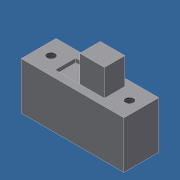
# Autodesk Inventor part: P1704_013_Switch
Saved by Autodesk Inventor 2019 (Build 230136000, 136)
## iProperties
Created: 2019-05-23
Part Number: P1704_013_Switch
Project: Nom Projet
Material: .
Description: Nom pièce
Document SubType Name: Modeling
Designer: Adel.KAHRIMANOVIC
Authority: brut Ø
Density: 0.001 g/cm^3
Appearance: Par défaut
Author: Adel.KAHRIMANOVIC
Material number: ---
Autodesk Inventor part; units mm, degrees
ref_plane "Plan YZ" through (0, 0, 0) normal (1, 0, 0) x (0, 1, 0)
ref_plane "Plan XZ" through (0, 0, 0) normal (0, 1, 0) x (-1, 0, 0)
ref_plane "Plan XY" through (0, 0, 0) normal (0, 0, 1) x (1, 0, 0)
sketch "Esquisse1" plane through (0, 0, 0) normal (0, 0, 1) x (1, 0, 0)
  line L0 (0, 0) -> (-25, 0)
  line L1 (-25, 0) -> (-25, 8.5)
  line L2 (-25, 8.5) -> (0, 8.5)
  line L3 (0, 8.5) -> (0, 0)
  dimension "d0" = 25
  dimension "d1" = 8.5
  constraints: 8 end point, 2 parallel, 1 horizontal, 1 perpendicular
  measures "d0" distance of L1.end L2.end
  measures "d1" distance between parallel lines of L0 L2
extrude "Extrusion1" add sketch "Esquisse1" along normal blind 11.5
sketch "Esquisse6" plane through (0, 0, 11.5) normal (0, 0, 1) x (1, 0, 0)
  line L0 (-18.5, 1.75) -> (-6.5, 1.75)
  line L1 (-6.5, 1.75) -> (-6.5, 6.75)
  line L2 (-6.5, 6.75) -> (-18.5, 6.75)
  line L3 (-18.5, 6.75) -> (-18.5, 1.75)
  line L4 (-6.5, 4.25) -> (0, 4.25) construction
  line L5 (0, 0) -> (0, 8.5) projected
  line L6 (-25, 4.25) -> (-18.5, 4.25) construction
  line L7 (-25, 8.5) -> (-25, 0) construction
  line L8 (-21.7955, 8.5) -> (-21.7955, 6.75) construction
  line L9 (-18.2379, 0) -> (-18.2379, 1.75) construction
  line L10 (-25, 0) -> (0, 0) construction
  line L11 (0, 8.5) -> (-25, 8.5) construction
  dimension "d4" = 5
  dimension "d5" = 12
  constraints: 16 end point, 4 midpoint, 4 point on line, 3 horizontal, 2 equal length, 2 parallel, 2 vertical, 1 collinear, 1 perpendicular
  measures "d4" distance between parallel lines of L2 L0
  measures "d5" distance of L1.end L2.end
extrude "Extrusion2" cut sketch "Esquisse6" against normal blind 1
sketch "Esquisse7" plane through (0, 0, 10.5) normal (0, 0, 1) x (1, 0, 0)
  line L0 (-6.5, 1.75) -> (-12.5, 1.75)
  line L1 (-12.5, 1.75) -> (-12.5, 6.75)
  line L2 (-12.5, 6.75) -> (-6.5, 6.75)
  line L3 (-6.5, 6.75) -> (-6.5, 1.75)
  line L4 (-6.5, 1.75) -> (-18.5, 1.75) projected
  line L5 (-18.5, 6.75) -> (-6.5, 6.75) projected
  line L6 (-6.5, 6.75) -> (-6.5, 1.75) projected
  point P0 (0, 0)
  dimension "d8" = 6
  constraints: 8 end point, 3 collinear, 2 parallel, 1 horizontal, 1 perpendicular
  measures "d8" distance of L1.end L2.end
extrude "Extrusion3" add sketch "Esquisse7" along normal blind 7.5
sketch "Esquisse8" plane through (0, 0, 11.5) normal (0, 0, 1) x (1, 0, 0)
  line L0 (-3, 4.354) -> (-3, 0.0702) construction
  line L1 (-3, 8.6378) -> (-3, 4.354) construction
  line L2 (0, 0) -> (0, 8.5) construction
  dimension "d18" = 3
  constraints: 4 end point, 2 vertical, 1 collinear
  measures "d18" distance from line of L2 L0.start
hole "Perçage1" at (-3, 4.354, 11.5) direction (0, 0, -1) diameter 2.013 end through all thread size "M2.5x0.45" class "6H" standard "ISO M"
sketch "Esquisse9" plane through (0, 0, 11.5) normal (0, 0, 1) x (1, 0, 0)
  line L0 (-25, 8.5) -> (-25, 0) projected
  line L1 (-22, 0.0375) -> (-22, 4.2687) construction
  line L2 (-22, 4.2687) -> (-22, 8.5) construction
  line L3 (0, 8.5) -> (-25, 8.5) construction
  point P0 (0, 0)
  dimension "d26" = 3
  constraints: 4 end point, 2 point on line, 1 collinear, 1 vertical
  measures "d26" distance from line of L0 L1.end
hole "Perçage2" at (-22, 4.2687, 11.5) direction (0, 0, -1) diameter 2.013 end through all thread size "M2.5x0.45" class "6H" standard "ISO M"
